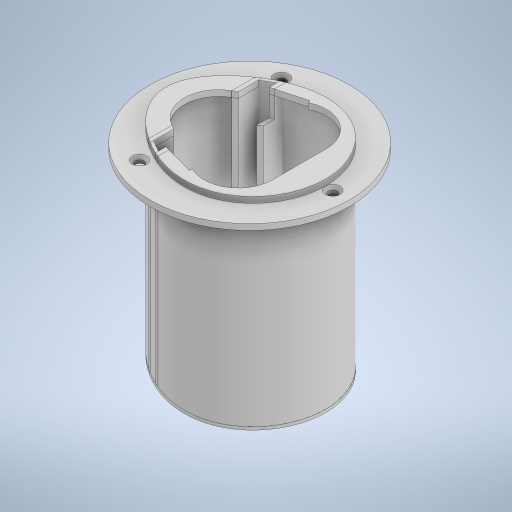
# Autodesk Inventor part: Akkuhalter_v2
Saved by Autodesk Inventor 2023 (Build 270158000, 158)
## iProperties
Created: 2022-06-27
Part Number: Akkuhalter_v2
Material: Generisch
Document SubType Name: Modeling
Designer: halal
Density: 1 g/cm^3
Appearance: Vorgabe
Author: halal
Autodesk Inventor part; units mm, degrees
ref_plane "YZ Plane" through (0, 0, 0) normal (1, 0, 0) x (0, 1, 0)
ref_plane "XZ Plane" through (0, 0, 0) normal (0, 1, 0) x (-1, 0, 0)
ref_plane "XY Plane" through (0, 0, 0) normal (0, 0, 1) x (1, 0, 0)
sketch "Vertikale Skizze" plane through (0, 0, 0) normal (0, 1, 0) x (-1, 0, 0)
  circle A0 centre (0, 0) radius 34
  line L0 (16.45, -10.1325) -> (0.55, -19.3124)
  line L1 (0.55, 19.3124) -> (16.45, 10.1325)
  line L2 (-17, 9.1799) -> (-17, -9.1799)
  arc A1 (16.45, -10.1325) -> (16.45, 10.1325) centre (10.6, 0) ccw
  arc A2 (-17, -9.1799) -> (0.55, -19.3124) centre (-5.3, -9.1799) ccw
  arc A3 (0.55, 19.3124) -> (-17, 9.1799) centre (-5.3, 9.1799) ccw
  line L3 (0.05, -41.02) -> (0.05, 48.4401) construction
  line L4 (-37.5507, 0) -> (39.6799, 0) construction
  line L5 (-38.2364, -40.7429) -> (-38.2364, 40.4504) construction
  line L6 (-38.2364, 40.4504) -> (37.6829, 40.4504) construction
  line L7 (37.6829, 40.4504) -> (37.6829, -40.7429) construction
  line L8 (37.6829, -40.7429) -> (-38.2364, -40.7429) construction
  spline S0 degree 5 poles (20.325, 13.6829) (15.6958, 17.9973) (5.2518, 24.5355) (-14.9508, 29.4884) (-38.3112, -0.6419) (-10.4044, -32.2661) (18.8724, -18.9452) (29.8471, -5.0698) (28.4631, 4.0846) (23.9161, 10.3359) (20.325, 13.6829) knots 0 0 0 0 0 0 0.219489 0.365814 0.538977 0.702893 0.82973 1 1 1 1 1 1
  line L9 (9.5539, 31.7924) -> (16.3479, 31.7924)
  line L10 (-38.2364, 40.4504) -> (37.6829, 40.4504)
  line L11 (37.6829, 40.4504) -> (37.6829, -40.7429)
  line L12 (37.6829, -40.7429) -> (-38.2364, -40.7429)
  line L13 (-38.2364, -40.7429) -> (-38.2364, 40.4504)
  line L14 (12.2019, 17.2626) -> (0.05, 20.5972)
  line L15 (0.05, 20.5972) -> (-0.2083, 19.6559)
  line L16 (-0.2083, 19.6559) -> (11.9436, 16.3214)
  line L17 (11.9436, 16.3214) -> (12.2019, 17.2626)
  line L18 (11.9436, 16.3214) -> (11.9436, 12.7342)
  line L19 (12.2019, -17.2626) -> (0.05, -20.5972)
  line L20 (0.05, -20.5972) -> (-0.2083, -19.6559)
  line L21 (-0.2083, -19.6559) -> (11.9436, -16.3214)
  line L22 (11.9436, -16.3214) -> (12.2019, -17.2626)
  line L23 (11.9436, -16.3214) -> (11.9436, -12.7342)
  circle A4 centre (13.5282, -24.3702) radius 1.5
  circle A5 centre (-28.3404, 0) radius 1.5
  circle A6 centre (13.5282, 23.998) radius 1.5
  spline S1 degree 5 poles (21.0068, 14.4144) (19.3432, 15.9647) (17.56, 17.3865) (15.6855, 18.6848) (11.6325, 21.0952) (7.2541, 22.8499) (4.9174, 23.5584) (0.0937, 24.5002) (-4.8181, 24.3352) (-7.2717, 23.9353) (-12.1002, 22.4446) (-16.3493, 19.7023) (-18.3039, 18.012) (-21.7886, 14.0941) (-24.1503, 9.4082) (-25.0337, 6.8792) (-26.112, 1.6418) (-25.7734, -3.6947) (-25.2406, -6.3253) (-23.5036, -11.3145) (-20.522, -15.6729) (-18.7736, -17.6178) (-14.8636, -20.9273) (-10.2175, -23.0752) (-7.8047, -23.8109) (-2.8953, -24.6004) (2.0573, -24.1715) (4.4707, -23.6821) (9.0484, -22.2818) (13.3232, -20.1289) (15.3227, -18.9285) (18.8853, -16.4447) (22.0725, -13.497) (23.453, -12.0336) (25.7692, -9.1441) (27.4659, -5.8622) (28.077, -4.2837) (28.8191, -1.0282) (28.5725, 2.3002) (28.1923, 3.9071) (26.9326, 7.241) (24.9447, 10.2115) (23.7289, 11.7038) (22.4111, 13.1062) (21.0068, 14.4144) knots 0 0 0 0 0 0 0.070887 0.070887 0.070887 0.146574 0.146574 0.146574 0.223108 0.223108 0.223108 0.302676 0.302676 0.302676 0.385239 0.385239 0.385239 0.467878 0.467878 0.467878 0.548441 0.548441 0.548441 0.626047 0.626047 0.626047 0.702248 0.702248 0.702248 0.774726 0.774726 0.774726 0.83728 0.83728 0.83728 0.889467 0.889467 0.889467 0.940167 0.940167 0.940167 1 1 1 1 1 1
  point P0 (34, 0)
  point P1 (-17, -29.4449)
  point P2 (-17, 29.4449)
  point P3 (27.6117, 0)
  point P4 (-24.8176, 0)
  point P5 (-6.1272, -22.9416)
  point P6 (20.325, -13.6829)
  point P7 (12.9509, 0)
  point P8 (0.05, 19.585)
  point P9 (0.05, -19.585)
  dimension "d64" = 1
  dimension "d3" = 68
  dimension "d4" = 11.7
  dimension "d207" = 3
  dimension "d208" = 3
  dimension "d209" = 3
  constraints: 40 end point, 12 point on line, 9 point on circle, 7 centre point, 7 symmetric about line, 6 tangent, 5 parallel, 3 vertical, 2 equal length, 2 equal radius, 2 horizontal, 2 perpendicular, 1 coincident, 10 other
  measures "d3" diameter of A0
  measures "d4" radius of A1
  measures "d207" diameter of A4
  measures "d208" diameter of A5
  measures "d209" diameter of A6
extrude "Hauptkörper oben" add sketch "Vertikale Skizze" along normal blind 2 contours L23 L21 A2 L0 | L22 L19 L20 A2 L21 | L1 A3 L16 L18 | L16 A3 L15 L14 L17 | S0 | S0
extrude "Hauptkörper unten" add sketch "Vertikale Skizze" against normal blind 66 contours S0 picked at (16.3449, 17.4878)
extrude "Bodenkörper" add sketch "Vertikale Skizze" against normal blind 1 separate body contours L0 A2 L21 L20 L2 A3 L15 L16 L1 A1 | L23 L21 A2 L0 | L22 L19 L20 A2 L21 | L1 A3 L16 L18 | A2 L20 L21 | L16 A3 L15 L14 L17 | L16 L15 A3 | S0 | S0
move or copy body "Boden" bodies to move or copy 2 copy no translate (0, -66, 0)
sketch "Akkuführungslasche vertikale Skizze" plane through (0, 2, 0) normal (0, 1, 0) x (1, 0, 0)
  line L0 (-16.3479, 31.7924) -> (-9.5539, 31.7924) projected
  line L1 (-16.3012, -31.7924) -> (-9.5539, -31.7924)
  line L2 (-9.5539, -31.7924) -> (-9.5539, 31.7924)
  line L3 (-9.5539, 31.7924) -> (-16.3012, 31.7924)
  line L4 (-16.3012, 31.7924) -> (-16.3012, -31.7924)
  line L5 (-16.3012, -31.7924) -> (-9.5539, 31.7924) construction
  line L6 (-9.5539, -31.7924) -> (-16.3012, 31.7924) construction
  line L7 (38.2191, 40.7482) -> (38.2191, -40.4058) construction
  line L8 (38.2191, -40.4058) -> (-37.6633, -40.4058) construction
  line L9 (-37.6633, -40.4058) -> (-37.6633, 40.7482) construction
  line L10 (-37.6633, 40.7482) -> (38.2191, 40.7482) construction
  line L11 (-10.9449, 22.7) -> (-14.9103, 22.7)
  line L12 (-14.9103, 22.7) -> (-14.9103, -22.7)
  line L13 (-14.9103, -22.7) -> (-10.9449, -22.7)
  line L14 (-10.9449, -22.7) -> (-10.9449, 22.7)
  line L15 (-10.9449, 22.7) -> (-14.9103, -22.7) construction
  line L16 (-14.9103, 22.7) -> (-10.9449, -22.7) construction
  point P0 (0, 0)
  point P1 (-12.9276, 0)
  constraints: 24 end point, 4 midpoint, 4 parallel, 2 horizontal, 2 perpendicular, 2 other
extrude "Akkuführungslasche" add sketch "Akkuführungslasche vertikale Skizze" against normal blind 68 separate body
extrude "Akkuführungslasche boolean" cut sketch "Vertikale Skizze" against normal blind 66 contours L0 A2 L21 L20 L2 A3 L15 L16 L1 A1 | A2 L20 L21 | L16 L15 A3 bodies 3
extrude "Extrusion13" cut sketch "Vertikale Skizze" along normal blind 2 contours L0 A2 L21 L20 L2 A3 L15 L16 L1 A1 | A2 L20 L21 | L16 L15 A3 bodies 3
extrude "Akkuführungslasche boolean außen" cut sketch "Vertikale Skizze" against normal blind 66 contours A0 | L10 L11 L12 L13 | A4 | A5 | A6 bodies 3
extrude "Extrusion15" cut sketch "Vertikale Skizze" along normal blind 2 contours A0 | L10 L11 L12 L13 | A4 | A5 | A6 bodies 3
extrude "Akkuführungslasche boolean hauptkörper" cut sketch "Akkuführungslasche vertikale Skizze" against normal blind 2 contours L14 L13 L12 L11 bodies 1
extrude "Hauptkörper Außenwand oben" add sketch "Vertikale Skizze" along normal blind 2 contours S0 picked at (16.3449, 17.4878) bodies 1
sketch "Skizze8" plane through (-0.8669, -67, -0.1153) normal (0, -1, 0) x (0.7315382, 0, 0.6818005)
  line L0 (55.893, 2.309) -> (-0.3724, -56.2203) construction
  line L1 (-0.3724, -56.2203) -> (-55.0998, -3.6098) construction
  line L2 (-55.0998, -3.6098) -> (1.1656, 54.9196) construction
  line L3 (1.1656, 54.9196) -> (55.893, 2.309) construction
  line L4 (-12.8447, 3.518) -> (-7.5672, -1.5554)
  line L5 (-7.5672, -1.5554) -> (-6.9076, -0.8692)
  line L6 (-6.9076, -0.8692) -> (-12.1851, 4.2042)
  line L7 (-12.1851, 4.2042) -> (-12.8447, 3.518)
  line L8 (-5.026, 11.6514) -> (0.2516, 6.578)
  line L9 (0.2516, 6.578) -> (0.8892, 7.2413)
  line L10 (0.8892, 7.2413) -> (-4.3883, 12.3147)
  line L11 (-4.3883, 12.3147) -> (-5.026, 11.6514)
  point P0 (0.7128, -0.5067)
  constraints: 16 end point, 4 parallel, 3 perpendicular, 2 point on line, 2 other
extrude "Kontaktlöcher" cut sketch "Skizze8" against normal blind 10 bodies 2
extrude "Akkuführungslasche boolean2" cut sketch "Vertikale Skizze" against normal blind 7 contours L23 L21 A2 L0 | L22 L19 L20 A2 L21 | L1 A3 L16 L18 | A2 L20 L21 | L16 A3 L15 L14 L17 | L16 L15 A3 bodies 1 3
extrude "Akkuführungslasche boolean3" cut sketch "Vertikale Skizze" along normal blind 2 contours L23 L21 A2 L0 | L22 L19 L20 A2 L21 | L1 A3 L16 L18 | A2 L20 L21 | L16 A3 L15 L14 L17 | L16 L15 A3 bodies 1 3
extrude "Halterungsebene" add sketch "Vertikale Skizze" against normal blind 2 separate body contours A0
chamfer "Schraubenlöcherabrundung" distance 1 angle 45 3 edges at (-12.0282, 0, -24.3702) (-12.0282, 0, 23.998) (29.8404, 0, 0)
equation "\"d3\" = Kreisradius"
equation "\"d4\" = Dreiecksabrundung"
equation "\"Dreiecksabrundung\" = 11.7"
equation "\"Dreieckskantenlänge\" = 57"
equation "\"Kreisradius\" = 68"
equation "\"Dreieckshöhe\" = 66"
equation "\"Wanddicke\" = 1"
equation "\"TestDreieckshöhe\" = 1"
equation "\"AußenkörperKreisRadius\" = 1"
equation "\"WagrechterAufsatzDicke\" = 2"
equation "\"KlippHöhe\" = 7"
equation "\"Lochdurchmesser\" = 3"
equation "\"BefestigungsDicke\" = 3"
equation "\"Phasendicke\" = 1"
